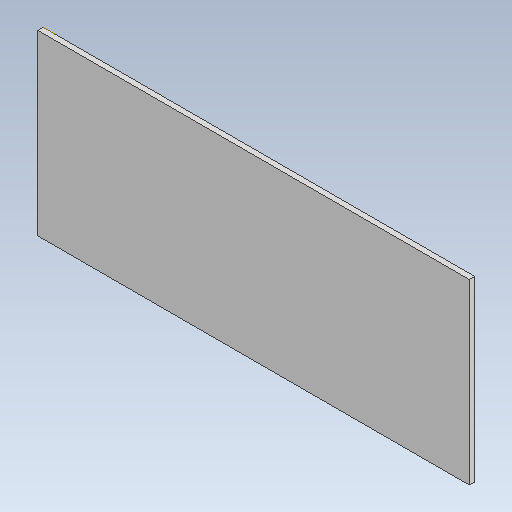
# Autodesk Inventor part: Pieza2
Saved by Autodesk Inventor 2020 (Build 240168000, 168)
## iProperties
Created: 2020-12-08
Part Number: Pieza2
Material: Genérico
Document SubType Name: Modeling
Designer: DanielAlvaradoPelaez
Density: 1 g/cm^3
Appearance: Valor por defecto
Author: DanielAlvaradoPelaez
Autodesk Inventor part; units mm, degrees
ref_plane "YZ Plane" through (0, 0, 0) normal (1, 0, 0) x (0, 1, 0)
ref_plane "XZ Plane" through (0, 0, 0) normal (0, 1, 0) x (-1, 0, 0)
ref_plane "XY Plane" through (0, 0, 0) normal (0, 0, 1) x (1, 0, 0)
ref_plane "Plano de trabajo1" through (-10, 10, 0) normal (0, 0, 1) x (1, 0, 0)
sketch "Boceto1" plane through (-10, 10, 0) normal (0, 0, 1) x (1, 0, 0)
  line L0 (0, 45) -> (800, 45)
  line L1 (800, 45) -> (800, -285)
  line L2 (800, -285) -> (0, -285)
  line L3 (0, -285) -> (0, 45)
  point P0 (10, -10)
  dimension "d0" = 800
  dimension "d1" = 330
  constraints: 8 end point, 2 parallel, 1 horizontal, 1 perpendicular
  measures "d0" distance of L1.end L2.end
  measures "d1" distance of L0.end L1.end
extrude "Extrusión1" add sketch "Boceto1" along normal blind 10
